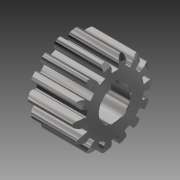
# Autodesk Inventor part: am-0034
Saved by Autodesk Inventor 2013 (Build 170138000, 138)
## iProperties
Shininess: 64.0
Length Units: 11272
Angle Units: 11279
Time Units: 11290
Mass Units: 11286
Length Display Precision: 3
Angle Display Precision: 2
Category: Drive Base Kit
Company: Autodesk Inc.
Created: 2012-12-15
Part Number: am-0034
Material: Steel, High Strength Low Alloy
Document SubType Name: Modeling
Designer: Autodesk Inc.
Catalog Web Link: http://www.andymark.com/product-p/am-0034.htm
Density: 7.84 g/cm^3
Mass: 20.3072 g
Surface Area: 23.8718 cm^2
Volume: 2.5902 cm^3
Vendor: AndyMark Inc.
Density: 7.84
Volumn: 6.736982259993864
Area: 35.592573078640946
PropertySet Name: Model Information
Control State: 0
Master: False
Checked Out: False
Author: Autodesk Inc.
Autodesk Inventor part; units mm, degrees
ref_plane "YZ Plane" through (0, 0, 0) normal (1, 0, 0) x (0, 1, 0)
ref_plane "XZ Plane" through (0, 0, 0) normal (0, 1, 0) x (-1, 0, 0)
ref_plane "XY Plane" through (0, 0, 0) normal (0, 0, 1) x (1, 0, 0)
sketch "Sketch2" plane through (6.35, 0, 0) normal (1, 0, 0) x (0, 0, -1)
  circle A0 centre (0, 0) radius 8.6068 construction
  arc A1 (1.9666, 9.9678) -> (-1.9666, 9.9678) centre (0, 0) ccw
  line L0 (0.9975, 8.8339) -> (3.0763, 8.0383) construction
  line L1 (0, 0) -> (0, 25.7198) construction
  circle A2 centre (0, 0) radius 8.89 projected
  arc A3 (1.9666, 9.9678) -> (0.8979, 7.5808) centre (3.0763, 8.0383) ccw
  arc A4 (-0.8979, 7.5808) -> (-1.9666, 9.9678) centre (-3.0763, 8.0383) ccw
  arc A5 (0.6275, 7.2755) -> (-0.6275, 7.2755) centre (0, 0) ccw
  line L2 (0, 0) -> (0, 42.0936) construction
  circle A6 centre (0, 0) radius 4 projected
  circle A7 centre (0, 0) radius 8.89 construction
  line L3 (-3.0763, 8.0383) -> (-0.9975, 8.8339) construction
  arc A8 (-0.8979, 7.5808) -> (-0.6275, 7.2755) centre (-0.6494, 7.5285) ccw
  arc A9 (0.6275, 7.2755) -> (0.8979, 7.5808) centre (0.6494, 7.5285) ccw
  dimension "d24" = 17.2137
  dimension "Root_Radius" = 7.3025
  dimension "d104" = 10.16
  dimension "Pitch_Diameter" = 17.78
  dimension "Tooth_Width" = 1.9949
  dimension "Root_Fillet" = 0.254
  dimension "d112" = 0.254
  constraints: 16 point on circle, 8 end point, 7 centre point, 6 coincident, 4 tangent, 1 point on line, 1 vertical, 6 other
  measures "Root_Radius" radius of A5
  measures "d104" radius of A1
  measures "Pitch_Diameter" diameter of A7
  measures "Tooth_Width" distance of L0.start L3.end
  measures "Root_Fillet" radius of A8
  measures "d112" radius of A9
sketch "Sketch1" plane through (0, 0, 0) normal (0, 0, 1) x (1, 0, 0)
  line L0 (6.35, 4) -> (6.35, 8.89)
  line L1 (5.6168, 10.16) -> (-5.6168, 10.16)
  line L2 (-6.35, 8.89) -> (-6.35, 4)
  line L3 (-6.35, 4) -> (6.35, 4)
  line L4 (6.35, 8.89) -> (5.6168, 10.16)
  line L5 (-6.35, 8.89) -> (-5.6168, 10.16)
  line L6 (-9.9568, 0) -> (9.9568, 0) projected
  line L7 (0, 0) -> (0, 27.4224) construction
  point P0 (0, 4)
  dimension "Bore_Radius" = 4
  dimension "Outside_Radius" = 10.16
  dimension "d77" = 8.89
  dimension "d108" = 30
  dimension "d109" = 30
  dimension "d110" = 12.7
  constraints: 14 end point, 3 vertical, 2 perpendicular, 1 coincident, 1 horizontal alignment, 1 midpoint, 1 point on line, 2 other
  measures "Bore_Radius" distance from line of point (0, 0) L3
  measures "Outside_Radius" distance from line of point (0, 0) L1
  measures "d77" distance from line of L6 L0.end
  measures "d108" angle of L5 L2
  measures "d109" angle of L4 L0
  measures "d110" distance of L2.end L0.start
revolve "Gear Blank" add sketch "Sketch1" angle 360 about axis through (-10, 0, 0) along (1, 0, 0)
extrude "Tooth Profile" cut sketch "Sketch2" against normal through all contours A3 A2 A4 A1 | A3 A9 A5 A8 A4 A2 picked at (0.0698, 8.3557)
pattern_circular "Circular Pattern" count 14 over 360 about axis through (0, 0, 0) along (1, 0, 0) of "Tooth Profile"
chamfer "Bore Chamfer Interior" distance 0.127 angle 45 1 edges at (6.35, -4, 0)
chamfer "Bore Chamfer Exterior" distance 0.127 angle 45 1 edges at (-6.35, -4, 0)
sketch "Sketch16" plane through (0, 0, 0) normal (1, 0, 0) x (0, 1, 0)
  line L0 (5, -1) -> (3, -1)
  line L1 (3, -1) -> (3, 1)
  line L2 (3, 1) -> (5, 1)
  line L3 (5, 1) -> (5, -1)
  line L4 (0, 0) -> (9.5781, 0) construction
  line L5 (0, 0) -> (0, 8.8774) construction
  dimension "d117" = 2
  dimension "d118" = 3
  constraints: 12 end point, 3 horizontal, 2 parallel, 2 perpendicular, 2 vertical, 1 other
  measures "d117" distance of L2.end L0.start
  measures "d118" distance between parallel lines of L5 L1
extrude "Key" cut sketch "Sketch16" along normal through all both and the other way through all
equation "\"Bore_Radius\" = 0.5 * Bore"
equation "\"Bore\" = 8"
equation "\"Pressure_Angle\" = 14.5deg"
equation "\"Hub_Diameter\" = 17.018"
equation "\"Hub_Thickness\" = 0.762"
equation "\"Key_Size\" = 2"
equation "\"Bore_Chamfer\" = 0.127"
equation "\"Face_Width\" = 12.7"
equation "\"Tooth_Chamfer\" = 30deg"
body "Solid1"
